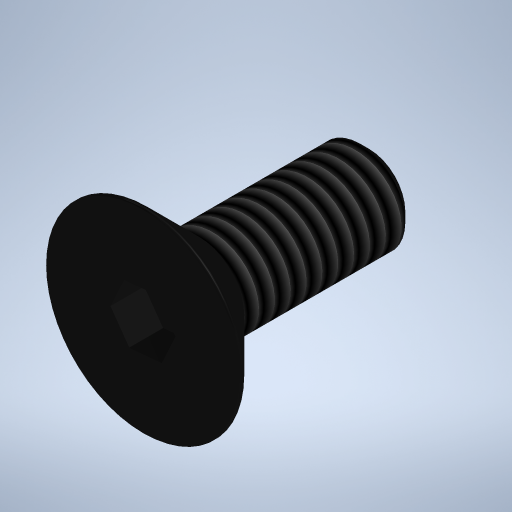
# Autodesk Inventor part: SCREW, FLAT HD, P, 12_9, M4X0_7X12MM
Saved by Autodesk Inventor 2024.2 (Build 282272000, 272)
## iProperties
Manager: 100-07244
Category: _
Shininess: 64.0
Created: 2013-09-09
Material: Generic
Document SubType Name: Modeling
Designer: keithl , Keith
Mass: 0.170884 g
Surface Area: 2.44459 cm^2
Volume: 0.170884 cm^3
Density: 1 g/cm^3
Checked By: 2FT8J
Engr Approved By: R
User Status: Released
Description: SCREW, FLAT HD, P, 12.9, M4X0.7X10MM
Mfg Approved By: Eric.Michaud
Part Number: SCREW, FLAT HD, P, 12_9, M4X0_7X12MM
Appearance: Glossy - Black
Density: 0.0
Volumn: 0.0
Area: 0.0
PropertySet Name: Model Information
Control State: 0
Master: False
Checked Out: False
CN_SERVICEABLE: _
CN_DETAILER: -
FIRST_DESCRIPTION: SCREW, FLAT HD, P, 12.9, M4X0.7X10MM
CN_MFG_NAME: -
STANDARDCLASSFLAG: R
CN_DESIGNER: Eric.Michaud
PTC_WM_ITERATION: 5
PTC_WM_ORGANIZATION_ID: CLWC
PTC_WM_LIFECYCLE: CLWC_CAD_LC
Author: -
Revision Number: 1
Keywords: -
Subject: _
Autodesk Inventor part; units mm, degrees
ref_plane "YZ Plane" through (0, 0, 0) normal (1, 0, 0) x (0, 1, 0)
ref_plane "XZ Plane" through (0, 0, 0) normal (0, 1, 0) x (-1, 0, 0)
ref_plane "XY Plane" through (0, 0, 0) normal (0, 0, 1) x (1, 0, 0)
sketch "Sketch1" plane through (0, 0, 0) normal (0, 0, 1) x (1, 0, 0)
  circle A0 centre (0, 0) radius 2
  dimension "Diameter" = 4
  constraints: 1 centre point
  measures "Diameter" diameter of A0
extrude "Extrusion1" add sketch "Sketch1" along normal blind 7.52
sketch "Sketch2" plane through (0, 0, 7.52) normal (0, 0, 1) x (1, 0, 0)
  circle A0 centre (0, 0) radius 2 projected
extrude "Extrusion2" add sketch "Sketch2" along normal blind 2.48 draft 45
sketch "Sketch3" plane through (0, 0, 10) normal (0, 0, 1) x (1, 0, 0)
  circle A0 centre (0, 0) radius 4.48 projected
  circle A1 centre (0, 0) radius 1.4434 construction
  line L0 (0.6042, 1.3108) -> (1.4373, 0.1322)
  line L1 (1.4373, 0.1322) -> (0.8331, -1.1787)
  line L2 (0.8331, -1.1787) -> (-0.6042, -1.3108)
  line L3 (-0.6042, -1.3108) -> (-1.4373, -0.1322)
  line L4 (-1.4373, -0.1322) -> (-0.8331, 1.1787)
  line L5 (-0.8331, 1.1787) -> (0.6042, 1.3108)
  dimension "Hex_Width" = 2.5
  constraints: 12 end point, 6 point on circle, 4 equal length, 1 centre point, 1 coincident
  measures "Hex_Width" distance between parallel lines of L0 L3
extrude "Extrusion3" cut sketch "Sketch3" against normal blind 1.5 contours L0 L1 L2 L3 L4 L5
thread "Thread1" size "M4x0.7" class "4g6g" standard "ANSI Metric M Profile" length 7.52
chamfer "Chamfer2" distance 0.4 angle 45 1 edges at (-2, 0, 0)
fillet "Fillet1" radius 0.1 1 edges at (-4.48, 0, 10)
equation "\"d10\" = Thread_Length"
equation "\"d13\" = Chamfer"
equation "\"Thread_Length\" = 7.52"
equation "\"Chamfer\" = 0.4"
body "Solid1"
